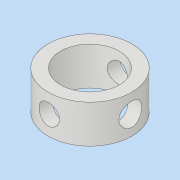
# Autodesk Inventor part: SpoolCarrageMagnetMount
Saved by Autodesk Inventor 2017 (Build 210142000, 142)
## iProperties
Created: 2018-04-12
Part Number: SpoolCarrageMagnetMount
Material: ABS Plastic
Document SubType Name: Modeling
Designer: Derek Wider
Density: 1.06 g/cm^3
Appearance: Smooth - White
Author: Derek Wider
Autodesk Inventor part; units mm, degrees
ref_plane "XZ Plane" through (0, 0, 0) normal (0, 1, 0) x (-1, 0, 0)
ref_plane "XY Plane" through (0, 0, 0) normal (0, 0, 1) x (1, 0, 0)
sketch "Sketch1" plane through (0, 0, 0) normal (0, 1, 0) x (-1, 0, 0)
  circle A0 centre (0, 0) radius 4.8895
  circle A1 centre (0, 0) radius 6.985
  dimension "d0" = 9.779
  dimension "d1" = 13.97
  constraints: 2 centre point, 2 coincident
  measures "d0" diameter of A0
  measures "d1" diameter of A1
extrude "Extrusion1" add sketch "Sketch1" along normal blind 6.35
ref_plane "Work Plane1" through (6.985, 0, 0) normal (1, 0, 0) x (0, 1, 0)
sketch "Sketch2" plane through (6.985, 0, 0) normal (1, 0, 0) x (0, 1, 0)
  circle A0 centre (3.175, 0) radius 1.905
  line L0 (0, -6.985) -> (6.35, -6.985) projected
  point P0 (0, 0)
  point P1 (3.175, -6.985)
  dimension "d4" = 3.81
  constraints: 1 centre point, 1 horizontal alignment, 1 midpoint, 1 vertical alignment
  measures "d4" diameter of A0
extrude "Extrusion2" cut sketch "Sketch2" against normal blind 6.35
sketch "Sketch3" plane through (0, 0, 0) normal (0, 0, 1) x (1, 0, 0)
  line L0 (-6.985, 0) -> (-6.985, 6.35) projected
  circle A0 centre (0, 3.175) radius 1.7145
  point P0 (0, 0)
  point P1 (-6.985, 3.175)
  dimension "d7" = 3.429
  constraints: 1 centre point, 1 horizontal alignment, 1 midpoint, 1 vertical alignment
  measures "d7" diameter of A0
extrude "Extrusion3" cut sketch "Sketch3" along normal through all both and the other way through all
body "Solid1"
